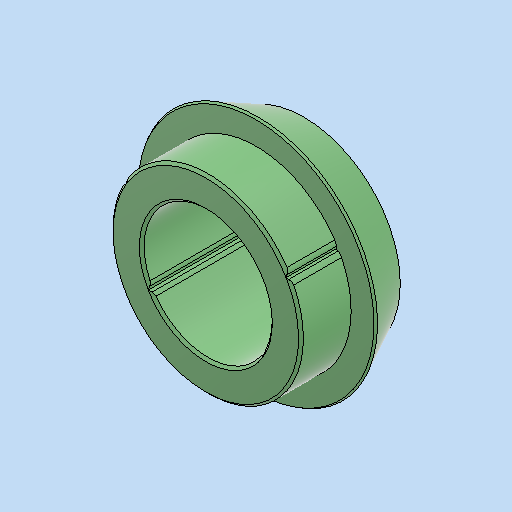
# Autodesk Inventor part: TouptekAdapterCylinder
Saved by Autodesk Inventor 2025 (Build 290162000, 162)
## iProperties
Created: 2025-02-20
Part Number: TouptekAdapterCylinder
Material: ABS Plastic
Document SubType Name: Modeling
Designer: kuzmin
Density: 1.06 g/cm^3
Appearance: Smooth - Dark Forest Green
Author: kuzmin
Autodesk Inventor part; units mm, degrees
ref_plane "YZ Plane" through (0, 0, 0) normal (1, 0, 0) x (0, 1, 0)
ref_plane "XZ Plane" through (0, 0, 0) normal (0, 1, 0) x (-1, 0, 0)
ref_plane "XY Plane" through (0, 0, 0) normal (0, 0, 1) x (1, 0, 0)
sketch "Sketch1" plane through (0, 0, 0) normal (0, 0, 1) x (1, 0, 0)
  circle A0 centre (0, 0) radius 15.95
  circle A1 centre (0, 0) radius 23.7
  dimension "d0" = 47.4
  dimension "d1" = 31.9
  constraints: 2 centre point, 2 coincident
  measures "d0" diameter of A1
  measures "d1" diameter of A0
extrude "Extrusion1" add sketch "Sketch1" along normal blind 25
sketch "Sketch2" plane through (0, 0, 0) normal (1, 0, 0) x (0, 1, 0)
  line L0 (23.7, 0) -> (23.7, 25) projected
  line L1 (23.7, 0) -> (30, 12.5)
  line L2 (30, 12.5) -> (23.7, 12.5)
  line L3 (0, 0) -> (0, 25)
  line L4 (23.7, 25) -> (-23.7, 25) projected
  point P0 (0, 12.5)
  dimension "d4" = 12.5
  dimension "d5" = 60
  constraints: 6 end point, 3 midpoint, 1 perpendicular
  measures "d4" distance from line of L2 L0.start
  measures "d5" diameter of L1.end point (0, 12.5)
revolve "Revolution1" add sketch "Sketch2" angle 360 about axis through (0, 0, 0) along (0, 0, 1)
sketch "Sketch3" plane through (0, 0, 25) normal (0, 0, 1) x (1, 0, 0)
  circle A0 centre (0, 0) radius 15.95 projected
  circle A1 centre (0, 0) radius 15.95 projected
  line L0 (-1, 15.9186) -> (0, 16.5819)
  line L1 (0, 16.5819) -> (1, 15.9186)
  line L2 (-1, 15.9186) -> (1, 15.9186)
  circle A2 centre (0, 0) radius 23.7 projected
  line L3 (20.0065, 12.7055) -> (19.9321, 11.5078)
  line L4 (19.9321, 11.5078) -> (21.0065, 10.9734)
  line L5 (20.0065, 12.7055) -> (21.0065, 10.9734)
  line L6 (20.5065, 11.8394) -> (0, 0) construction
  line L7 (0, 0) -> (0, 16.5819) construction
  dimension "d11" = 1.2
  dimension "d12" = 2
  dimension "d16" = 1.2
  dimension "d17" = 2
  dimension "d26" = 60
  constraints: 16 end point, 4 point on circle, 1 equal length, 1 horizontal, 1 midpoint, 1 point on line, 1 vertical, 1 vertical alignment
  measures "d11" distance of L0.end L1.end
  measures "d12" distance of L0.start L1.end
  measures "d16" distance of L3.start L3.end
  measures "d17" distance of L3.start L4.end
  measures "d26" angle of L7 L6
extrude "Extrusion2" cut sketch "Sketch3" against normal through all contours L2 A0 | A0 L0 L1 picked at (-0.1112, 15.9279)
extrude "Extrusion3" cut sketch "Sketch3" against normal up to surface (12.5 mm away) contours L5 A2 | L4 L3 L5
pattern_circular "Circular Pattern1" count 3 over 360 about axis through (0, 0, 0) along (0, 0, 1) of "Extrusion3"
pattern_circular "Circular Pattern2" count 3 over 360 about axis through (0, 0, 0) along (0, 0, 1) of "Extrusion2"
chamfer "Chamfer1" distance 0.6 angle 45 11 edges at (-13.8131, 7.975, 0) (0, -15.95, 0) (13.8131, 7.975, 0) (0, -23.7, 0) (0, -30, 12.5) (20.5248, -11.85, 25) (0, 23.7, 25) (-20.5248, -11.85, 25) (-13.8131, 7.975, 25) (0, -15.95, 25) (13.8131, 7.975, 25)
fillet "Fillet1" radius 2 12 edges at (-1, 15.9186, 12.5) (1, 15.9186, 12.5) (20.0065, 12.7055, 18.45) (21.0065, 10.9734, 18.45) (-1, -23.6789, 18.45) (1, -23.6789, 18.45) (-20.0065, 12.7055, 18.45) (-21.0065, 10.9734, 18.45) (-13.2859, -8.8253, 12.5) (-14.2859, -7.0933, 12.5) (13.2859, -8.8253, 12.5) (14.2859, -7.0933, 12.5)
body "Solid1"
